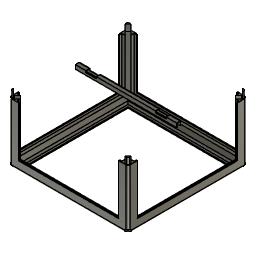
LEDCube (Autodesk Fusion 360 design; units mm, degrees)
Autodesk Fusion 360 part; units mm, degrees
note: some values were not read from the file. Set by a fixed rule: which face or edge a step refers to.
sketch "Initial Square" plane through (0, 0, 0) normal (0, 0, 1) x (1, 0, 0)
  line L0 (-56.3284, 56.3284) -> (56.3284, 56.3284)
  line L1 (56.3284, 56.3284) -> (56.3284, -56.3284)
  line L2 (56.3284, -56.3284) -> (-56.3284, -56.3284)
  line L3 (-56.3284, -56.3284) -> (-56.3284, 56.3284)
  line L4 (-56.3284, 56.3284) -> (56.3284, -56.3284) construction
  line L5 (56.3284, 56.3284) -> (-56.3284, -56.3284) construction
  dimension "d1" = 112.6569
  dimension "d2" = 112.6569
  constraint horizontal L0
  constraint perpendicular L0 L1
  constraint parallel L0 L2
  constraint parallel L1 L3
  constraint coincident L4 origin
  constraint coincident L5 origin
  measures "d1" distance of L1.end L2.end
  measures "d2" distance of L0.end L1.end
extrude "Extrude1" add sketch "Initial Square" along normal mid plane 112.6569 makes body 1
shell "Shell1" thickness 4 removed faces 0 bodies 1
chamfer "Chamfer1" distance 2.83 angle 45 12 edges at (0, -52.3284, 52.3284) (-52.3284, -52.3284, 0) (52.3284, -52.3284, 0) (52.3284, 0, 52.3284) (52.3284, 52.3284, 0) (0, 52.3284, -52.3284) (52.3284, 0, -52.3284) (0, -52.3284, -52.3284) (-52.3284, 0, -52.3284) (-52.3284, 0, 52.3284) (-52.3284, 52.3284, 0) (0, 52.3284, 52.3284) on bodies 1
sketch "Square cutout" plane through (0, -56.3284, 0) normal (0, -1, 0) x (1, 0, 0)
  line L0 (56.3284, -56.3284) -> (56.3284, 56.3284)
  line L1 (56.3284, 56.3284) -> (-56.3284, 56.3284)
  line L2 (-56.3284, 56.3284) -> (-56.3284, -56.3284)
  line L3 (-56.3284, -56.3284) -> (56.3284, -56.3284)
  line L4 (47.5, -47.5) -> (-47.5, -47.5)
  line L5 (-47.5, -47.5) -> (-47.5, 47.5)
  line L6 (-47.5, 47.5) -> (47.5, 47.5)
  line L7 (47.5, 47.5) -> (47.5, -47.5)
  line L8 (47.5, -47.5) -> (-47.5, 47.5) construction
  line L9 (-47.5, -47.5) -> (47.5, 47.5) construction
  dimension "d7" = 95
  dimension "d8" = 95
  constraint horizontal L4
  constraint perpendicular L4 L5
  constraint parallel L4 L6
  constraint parallel L5 L7
  constraint coincident L8 origin
  constraint coincident L9 origin
  measures "d7" distance of L5.end L6.end
  measures "d8" distance of L4.end L5.end
extrude "Extrude2" cut sketch "Square cutout" against normal through all contours L4 L5 L6 L7 bodies 1
extrude "Extrude3" cut 1 faces at (48.8323, -52.3284, -15.8333) along direction (0, -1, 0) blind 3 on bodies 1 bodies 1
pattern_circular "C-Pattern1" count 4 over 360 about axis through (0, 0, 1.75) along (0, 0, 1) of "Extrude2", "Extrude3"
pattern_circular "C-Pattern2" count 4 over 360 about axis through (1.75, 0, 0) along (1, 0, 0) of "Extrude2", "Extrude3"
fillet "Fillet1" radius 2 12 edges at (56.3284, -56.3284, 0) (56.3284, 0, 56.3284) (0, -56.3284, 56.3284) (-56.3284, -56.3284, 0) (0, 56.3284, 56.3284) (-56.3284, 0, 56.3284) (56.3284, 56.3284, 0) (-56.3284, 56.3284, 0) (0, 56.3284, -56.3284) (-56.3284, 0, -56.3284) (0, -56.3284, -56.3284) (56.3284, 0, -56.3284) on bodies 1
extrude "Extrude channels" cut 1 faces at (-16.4995, -50.4418, -51.3851) along direction (0, -0.707107, -0.707107) blind 4 on bodies 1 bodies 1
pattern_circular "C-Pattern9" count 4 over 360 about axis through (1.75, 0, 0) along (1, 0, 0) of "Extrude channels"
extrude "Extrude16" cut 1 faces at (-50.4418, -16.4995, -51.3851) along direction (-0.707107, 0, -0.707107) blind 4 on bodies 1 bodies 1
pattern_circular "C-Pattern10" count 4 over 360 about axis through (0, 1.75, 0) along (0, 1, 0) of "Extrude16"
extrude "Extrude17" cut 1 faces at (50.4418, 51.3851, -16.4995) along direction (0.707107, 0.707107, 0) blind 4 on bodies 1 bodies 1
pattern_circular "C-Pattern11" count 4 over 360 about axis through (0, 0, 1.75) along (0, 0, 1) of "Extrude17"
delete_face "DeleteFace1" 4 faces at (49.4984, -53.2707, 52.3274) (50.4418, -50.4418, 50.4418) (52.3279, -49.4984, 51.3846) (52.3279, -51.3846, 49.4984) on bodies 1
delete_face "DeleteFace2" 4 faces at (49.4984, 52.3274, 53.2707) (52.3274, 49.4984, 53.2707) (50.4418, 50.4418, 50.4418) (52.3274, 53.2707, 49.4984) on bodies 1
delete_face "DeleteFace3" 4 faces at (-52.3274, 49.4984, 53.2707) (-49.4984, 52.3274, 53.2707) (-50.4418, 50.4418, 50.4418) (-51.3846, 52.3279, 49.4984) on bodies 1
delete_face "DeleteFace4" 4 faces at (-49.4984, -51.3846, 52.3279) (-50.4418, -50.4418, 50.4418) (-53.2707, -49.4984, 52.3274) (-52.3279, -51.3846, 49.4984) on bodies 1
delete_face "DeleteFace5" 4 faces at (-50.4418, -50.4418, -50.4418) (-52.3279, -49.4984, -51.3846) (-51.3846, -52.3279, -49.4984) (-49.4984, -52.3274, -53.2707) on bodies 1
delete_face "DeleteFace6" 4 faces at (-49.4984, 51.3846, -52.3279) (-52.3274, 53.2707, -49.4984) (-50.4418, 50.4418, -50.4418) (-53.2707, 49.4984, -52.3274) on bodies 1
delete_face "DeleteFace7" 4 faces at (53.2707, 52.3274, -49.4984) (50.4418, 50.4418, -50.4418) (49.4984, 53.2707, -52.3274) (51.3846, 49.4984, -52.3279) on bodies 1
delete_face "DeleteFace8" 4 faces at (49.4984, -52.3279, -51.3846) (52.3279, -51.3846, -49.4984) (50.4418, -50.4418, -50.4418) (53.2707, -49.4984, -52.3274) on bodies 1
ref_plane "WorkPlane1" through (52.3284, -49.4984, -49.4984) normal (0.57735, -0.57735, -0.57735) x (0.707107, 0.707107, 0)
sketch "Wire hole" plane through (52.3284, -49.4984, -49.4984) normal (0.57735, -0.57735, -0.57735) x (0.707107, 0.707107, 0)
  circle A0 centre (-2.0011, -1.1553) radius 2.3107 construction
  circle A1 centre (-2.0011, -1.1553) radius 2
  point P0 (-2.0011, -3.466)
  point P1 (-4.0022, 0)
  dimension "d95" = 4
  constraint coincident origin A0
  constraint coincident P1 A0
  constraint coincident P0 A0
  constraint concentric A0 A1
  measures "d95" diameter of A1
extrude "Extrude19" cut sketch "Wire hole" along normal through all bodies 1
fillet "Fillet5" radius 0.2 6 edges at (55.7426, -53.2932, -55.7426) (53.8789, -53.8789, -56.3284) (53.2932, -55.7426, -55.7426) (53.8789, -56.3284, -53.8789) (55.7426, -55.7426, -53.2932) (56.3284, -53.8789, -53.8789) on bodies 1
split "Split1" by plane through (0, 0, 0) normal (0, 0, 1) bodies 1 makes body 2 at (-15.8333, 52.0523, 56.3284)
copy_body "Body->Comp1" bodies 1 removing the originals makes body 3 in component "Bottom"
copy_body "Body->Comp2" bodies 2 removing the originals makes body 4 in component "Top"
sketch "Insert" plane through (0, 0, 0) normal (0, 0, 1) x (1, 0, 0)
  line L0 (49.5, 2) -> (-49.5, 2)
  line L1 (-49.5, 2) -> (-49.5, -2)
  line L2 (-49.5, -2) -> (49.5, -2)
  line L3 (49.5, -2) -> (49.5, 2)
  line L4 (49.5, 2) -> (-49.5, -2) construction
  line L5 (-49.5, 2) -> (49.5, -2) construction
  dimension "d98" = 99
  dimension "d99" = 4
  constraint horizontal L0
  constraint perpendicular L0 L1
  constraint parallel L0 L2
  constraint parallel L1 L3
  constraint coincident L4 origin
  constraint coincident L5 origin
  measures "d98" distance of L1.end L2.end
  measures "d99" distance of L0.end L1.end
sketch "Insert (2)" plane through (0, 0, 0) normal (0, 0, 1) x (1, 0, 0) in component "Insert"
  line L0 (48, -1.9) -> (-48, -1.9)
  line L1 (-48, -1.9) -> (-48, 1.9)
  line L2 (-48, 1.9) -> (48, 1.9)
  line L3 (48, 1.9) -> (48, -1.9)
  line L4 (48, -1.9) -> (-48, 1.9) construction
  line L5 (-48, -1.9) -> (48, 1.9) construction
  dimension "d103" = 96
  dimension "d104" = 3.8
  constraint horizontal L0
  constraint perpendicular L0 L1
  constraint parallel L0 L2
  constraint parallel L1 L3
  constraint coincident L4 origin
  constraint coincident L5 origin
  measures "d103" distance of L1.end L2.end
  measures "d104" distance of L0.end L1.end
extrude "Extrude1'" add sketch "Insert (2)" along normal blind 3.8 separate body makes body 5 in component "Insert"
sketch "Channel" plane through (48, 0, 0) normal (1, 0, 0) x (0, 1, 0) in component "Insert"
  line L0 (-1.9, 0) -> (1.9, 0)
  line L1 (1.9, 0) -> (1.9, 3.8)
  line L2 (1.9, 3.8) -> (-1.9, 3.8)
  line L3 (-1.9, 3.8) -> (-1.9, 0)
  line L4 (1.5, 0) -> (1.5, 3.4)
  line L5 (1.5, 3.4) -> (-1.5, 3.4)
  line L6 (-1.5, 3.4) -> (-1.5, 0)
  dimension "d107" = -0.4
extrude "Extrude2'" cut sketch "Channel" against normal through all contours L0 L4 L5 L6 bodies 5 in component "Insert"
sketch "Solder hole" plane through (0, 0, 3.8) normal (0, 0, 1) x (-1, 0, 0) in component "Insert"
  line L0 (-48, -1.9) -> (48, -1.9)
  line L1 (48, -1.9) -> (48, 1.9)
  line L2 (48, 1.9) -> (-48, 1.9)
  line L3 (-48, 1.9) -> (-48, -1.9)
  line L4 (48, -1.9) -> (38, -1.9) construction
  line L5 (38, -1.9) -> (28, -1.9)
  line L6 (28, -1.9) -> (28, 1.9)
  line L7 (28, 1.9) -> (38, 1.9)
  line L8 (38, 1.9) -> (38, -1.9)
  dimension "d109" = 10
  dimension "d110" = 10
  constraint coincident L0.end L1.start
  constraint perpendicular L1 L4
  constraint horizontal L5
  constraint vertical L6
  constraint horizontal L7
  constraint vertical L8
  constraint equal L1 L8
  measures "d109" distance of L0.end L4.end
  measures "d110" distance of L4.end L5.end
extrude "Extrude3'" cut sketch "Solder hole" against normal blind 1.6 contours L0 L2 L5 L6 L7 L8 bodies 5 in component "Insert"
mirror "Mirror1" about plane through (0, 0, 0) normal (1, 0, 0) of "Extrude3'" in component "Insert"
sketch "Sketch1" plane through (0, 0, 0) normal (0, 0, 1) x (-1, 0, 0) in component "Bottom"
  arc A0 (54.3284, -56.3284) -> (56.3284, -54.3284) centre (54.3284, -54.3284) ccw
  line L0 (56.3284, -54.3284) -> (56.3284, -47.5)
  line L1 (56.3284, -47.5) -> (55.3284, -47.5)
  line L2 (55.3284, -47.5) -> (55.3284, -49.4984)
  line L3 (55.3284, -49.4984) -> (52.3284, -49.4984)
  line L4 (52.3284, -49.4984) -> (55.1569, -52.3269)
  line L5 (55.1569, -52.3269) -> (52.3269, -55.1569)
  line L6 (52.3269, -55.1569) -> (49.4984, -52.3284)
  line L7 (49.4984, -52.3284) -> (49.4984, -55.3284)
  line L8 (49.4984, -55.3284) -> (47.5, -55.3284)
  line L9 (47.5, -55.3284) -> (47.5, -56.3284)
  line L10 (47.5, -56.3284) -> (54.3284, -56.3284)
  arc A1 (54.3284, -55.6284) -> (55.6284, -54.3284) centre (54.3284, -54.3284) ccw
  line L11 (55.6518, -52.8218) -> (52.8218, -55.6518)
  line L12 (55.6284, -54.3284) -> (55.6284, -52.8218)
  line L13 (55.6284, -52.8218) -> (55.6518, -52.8218)
  line L14 (54.3284, -55.6284) -> (52.8218, -55.6284)
  line L15 (52.8218, -55.6284) -> (52.8218, -55.6518)
  dimension "d116" = -0.7
  dimension "d117" = -0.7
  constraint tangent A1 L12
  constraint perpendicular L12 L13
  constraint tangent A1 L14
  constraint parallel L12 L15
extrude "Extrude1''" add sketch "Sketch1" along normal blind 6 contours A1 L11 L12 L14 bodies 3 in component "Bottom"
pattern_circular "C-Pattern1'" count 4 over 360 about axis through (0, 0, 1.75) along (0, 0, 1) of "Extrude1''" in component "Bottom"
sketch "Sketch1 (2)" plane through (0, 0, 0) normal (0, 0, -1) x (1, 0, 0) in component "Top"
  arc A0 (-56.3284, -54.3284) -> (-54.3284, -56.3284) centre (-54.3284, -54.3284) ccw
  line L0 (-54.3284, -56.3284) -> (-47.5, -56.3284)
  line L1 (-47.5, -56.3284) -> (-47.5, -55.3284)
  line L2 (-47.5, -55.3284) -> (-49.4984, -55.3284)
  line L3 (-49.4984, -55.3284) -> (-49.4984, -52.3284)
  line L4 (-49.4984, -52.3284) -> (-52.3269, -55.1569)
  line L5 (-52.3269, -55.1569) -> (-55.1569, -52.3269)
  line L6 (-55.1569, -52.3269) -> (-52.3284, -49.4984)
  line L7 (-52.3284, -49.4984) -> (-55.3284, -49.4984)
  line L8 (-55.3284, -49.4984) -> (-55.3284, -47.5)
  line L9 (-55.3284, -47.5) -> (-56.3284, -47.5)
  line L10 (-56.3284, -47.5) -> (-56.3284, -54.3284)
  arc A1 (55.6284, 54.3284) -> (54.3284, 55.6284) centre (54.3284, 54.3284) ccw
  line L11 (54.3284, 55.6284) -> (52.8452, 55.6284)
  line L12 (52.8452, 55.6284) -> (55.6284, 52.8452)
  line L13 (55.6284, 52.8452) -> (55.6284, 54.3284)
  line L14 (52.3624, 55.8284) -> (55.8284, 52.3624)
  line L15 (55.8284, 52.3624) -> (55.8284, 54.3284)
  arc A2 (55.8284, 54.3284) -> (54.3284, 55.8284) centre (54.3284, 54.3284) ccw
  line L16 (54.3284, 55.8284) -> (52.3624, 55.8284)
  dimension "d127" = 0.2
extrude "Extrude3''" cut sketch "Sketch1 (2)" against normal blind 6.4 contours A1 L11 L12 L13 | L14 L15 A2 L16 bodies 4 in component "Top"
pattern_circular "C-Pattern2'" count 4 over 360 about axis through (0, 0, 1.75) along (0, 0, 1) of "Extrude3''" in component "Top"
component "Bottom" placed x (1, 0, 0) y (0, 1, 0) z (0, 0, 1) at (0, 0, 0)
component "Top" placed x (1, 0, 0) y (0, 1, 0) z (0, 0, 1) at (0, 0, 0)
component "Insert" placed x (1, 0, 0) y (0, 1, 0) z (0, 0, 1) at (0, 0, 0)
equation "d1 = Cubesize"
equation "d2 = Cubesize"
equation "d3 = Cubesize / 2"
equation "Cubesize = ( 2 * ( sqrt(8) + 4 + 2 ) ) * 1 mm + 95 mm"
